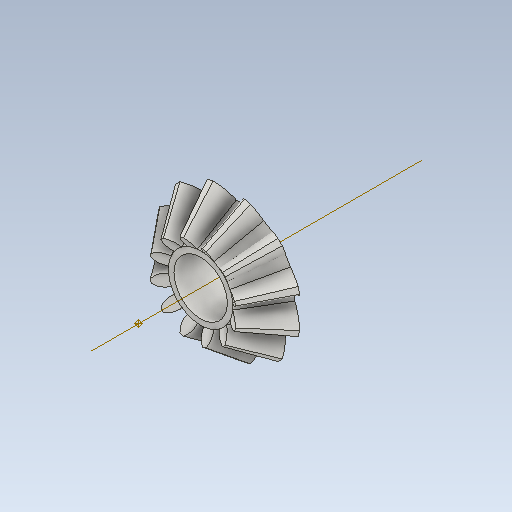
# Autodesk Inventor part: Коническая зубчатая передача12_КОПИЯ1
Saved by Autodesk Inventor 2020 (Build 240168000, 168)
## iProperties
Created: 2021-02-28
Part Number: Коническая зубчатая передача12_КОПИЯ1
Material: Steel, Mild
Document SubType Name: Modeling
Designer: Антон
Categories: <?xml version="1.0" encoding="UTF-16"?> <MemberInstance><Categories><FamilyTemplate><FamilyTemplateParameter ValueType="xs:double" Id="1" ObjectReferenceKey="da_z" ObjectType="kUserParameterObject"/><FamilyTemplateParameter ValueType="xs:double" Id="2" ObjectReferenceKey="da_b" ObjectType="kUserParameterObject"/><FamilyTemplateParameter ValueType="xs:double" Id="3" ObjectReferenceKey="da_beta" ObjectType="kUserParameterObject"/><FamilyTemplateParameter ValueType="xs:double" Id="4" ObjectReferenceKey="da_dae" ObjectType="kUserParameterObject"/><FamilyTemplateParameter ValueType="xs:double" Id="5" ObjectReferenceKey="da_ve" ObjectType="kUserParameterObject"/><FamilyTemplateParameter ValueType="xs:double" Id="6" ObjectReferenceKey="da_omega" ObjectType="kUserParameterObject"/><FamilyTemplateParameter ValueType="xs:string" Id="7" ObjectReferenceKey="EAIAABAAAAAAHwAAAAAAAIAAAAAAAAAA" ObjectType="83914240" SubObjectId="SurfaceGeometry"/></FamilyTemplate><ParamToTemplateMap><ParamToTemplate CategoryParameter="//CategoryParameter[@InternalName='046C89C9-8512-4d59-83FE-43B91F4F132A']" TemplateParameter="1"/><ParamToTemplate CategoryParameter="//CategoryParameter[@InternalName='2552DF32-E462-4b46-AEBF-C6C7768E72AC']" TemplateParameter="2"/><ParamToTemplate CategoryParameter="//CategoryParameter[@InternalName='C9EE641D-15FC-4fae-A226-E94C4372FDD7']" TemplateParameter="3"/><ParamToTemplate><ParamToTemplate CategoryParameter="//CategoryParameter[@InternalName='00B6519A-459B-49c7-AD84-2E56D39A5744']" ConstantValue="0.000000"/></ParamToTemplate><ParamToTemplate><ParamToTemplate CategoryParameter="//CategoryParameter[@InternalName='04B31F0E-C7A6-4894-AA32-9629BEFACF47']" ConstantValue="1.000000"/></ParamToTemplate><ParamToTemplate><ParamToTemplate CategoryParameter="//CategoryParameter[@InternalName='43CBEC2E-7847-49e7-A936-2F7889FCB2D9']" ConstantValue="0.200000"/></ParamToTemplate><ParamToTemplate><ParamToTemplate CategoryParameter="//CategoryParameter[@InternalName='B1EFC894-105D-4ebd-86BF-FA20ED196853']" ConstantValue="0.300000"/></ParamToTemplate><ParamToTemplate><ParamToTemplate CategoryParameter="//CategoryParameter[@InternalName='51175063-3D10-4879-93E8-6246FE8B403D']" ConstantValue="2060000000.000000"/></ParamToTemplate><ParamToTemplate><ParamToTemplate CategoryParameter="//CategoryParameter[@InternalName='A3A52E27-4454-46a9-B0BD-C932399B70AF']" ConstantValue="0.300000"/></ParamToTemplate><ParamToTemplate CategoryParameter="//CategoryParameter[@InternalName='2A200944-5A8C-41ca-B96E-8520D2E510F1']" TemplateParameter="4"/><ParamToTemplate><ParamToTemplate CategoryParameter="//CategoryParameter[@InternalName='1A637F62-92C8-44bc-B81F-10802510B579']" ConstantValue="0.818045"/></ParamToTemplate><ParamToTemplate CategoryParameter="//CategoryParameter[@InternalName='B52DD4BE-6863-48fb-BF58-89EF6F9EC65C']" TemplateParameter="5"/><ParamToTemplate><ParamToTemplate CategoryParameter="//CategoryParameter[@InternalName='3956BFF2-84D2-457d-93C2-9B0613DEBA67']" ConstantValue="0.510523"/></ParamToTemplate><ParamToTemplate CategoryParameter="//CategoryParameter[@InternalName='739CFA02-461B-4bf8-8049-181FCAD8B28F']" TemplateParameter="6"/><ParamToTemplate><ParamToTemplate CategoryParameter="//CategoryParameter[@InternalName='A27E999F-E2CE-4481-8A2A-EBF499C4C3C5']" ConstantValue="0.000000"/></ParamToTemplate><ParamToTemplate><ParamToTemplate CategoryParameter="//CategoryParameter[@InternalName='9E1B4470-B2D3-4ff1-B813-535BB4CDF51A']" ConstantValue="3520000.000000"/></ParamToTemplate><ParamToTemplate><ParamToTemplate CategoryParameter="//CategoryParameter[@InternalName='F8452263-BFF6-458c-9FB1-07C4B99E95CD']" ConstantValue="11400000.000000"/></ParamToTemplate><ParamToTemplate><ParamToTemplate CategoryParameter="//CategoryParameter[@InternalName='3E3BB259-FD49-497f-8171-6EBC954A3479']" ConstantValue="2.000000"/></ParamToTemplate><ParamToTemplate CategoryParameter="//CategoryParameter[@InternalName='27C3BAF2-7550-4e4b-AE2C-0DB134B7D9B7']" TemplateParameter="7"/></ParamToTemplateMap><Category DisplayName="Gear" InternalName="DC85795E-93AB-48d5-8EEE-5A27447B64BD" Mnemonic="Gear"><CategoryParameter DisplayName="z" InternalName="046C89C9-8512-4d59-83FE-43B91F4F132A" Mnemonic="z"/><CategoryParameter DisplayName="b" InternalName="2552DF32-E462-4b46-AEBF-C6C7768E72AC" Mnemonic="b"/><CategoryParameter DisplayName="||b|" InternalName="C9EE641D-15FC-4fae-A226-E94C4372FDD7" Mnemonic="beta"/><CategoryParameter DisplayName="x" InternalName="00B6519A-459B-49c7-AD84-2E56D39A5744" Mnemonic="x"/><CategoryParameter DisplayName="a*" InternalName="04B31F0E-C7A6-4894-AA32-9629BEFACF47" Mnemonic="a"/><CategoryParameter DisplayName="c*" InternalName="43CBEC2E-7847-49e7-A936-2F7889FCB2D9" Mnemonic="c"/><CategoryParameter DisplayName="r|.f|*" InternalName="B1EFC894-105D-4ebd-86BF-FA20ED196853" Mnemonic="rf"/><CategoryParameter DisplayName="E" InternalName="51175063-3D10-4879-93E8-6246FE8B403D" Mnemonic="E"/><CategoryParameter DisplayName="||m|" InternalName="A3A52E27-4454-46a9-B0BD-C932399B70AF" Mnemonic="mi"/><Category DisplayName="BevelGear" InternalName="0C98F69A-0C2B-4791-B2FE-7691BB227E77" Mnemonic="BevelGear"><CategoryParameter DisplayName="d|.ae|" InternalName="2A200944-5A8C-41ca-B96E-8520D2E510F1" Mnemonic="dae"/><CategoryParameter DisplayName="d|.ai|" InternalName="1A637F62-92C8-44bc-B81F-10802510B579" Mnemonic="dai"/><CategoryParameter DisplayName="J|.e|" InternalName="B52DD4BE-6863-48fb-BF58-89EF6F9EC65C" Mnemonic="ve"/><CategoryParameter DisplayName="J|.i|" InternalName="3956BFF2-84D2-457d-93C2-9B0613DEBA67" Mnemonic="vi"/><CategoryParameter DisplayName="||S|" InternalName="739CFA02-461B-4bf8-8049-181FCAD8B28F" Mnemonic="omega"/><CategoryParameter DisplayName="x|.t|" InternalName="A27E999F-E2CE-4481-8A2A-EBF499C4C3C5" Mnemonic="xt"/><CategoryParameter DisplayName="||s||.Flim|" InternalName="9E1B4470-B2D3-4ff1-B813-535BB4CDF51A" Mnemonic="sFlim"/><CategoryParameter DisplayName="||s||.Hlim|" InternalName="F8452263-BFF6-458c-9FB1-07C4B99E95CD" Mnemonic="sHlim"/><CategoryParameter DisplayName="тип" InternalName="3E3BB259-FD49-497f-8171-6EBC954A3479" Mnemonic="type"/><CategoryParameter DisplayName="PitchDiameter" InternalName="27C3BAF2-7550-4e4b-AE2C-0DB134B7D9B7" Mnemonic="IDS_PITCHDIAM"/></Category></Category></Categories></MemberInstance>
Mass: 60.9118 g
Surface Area: 34.3074 cm^2
Volume: 7.7496 cm^3
Density: 7.85 g/cm^3
Appearance: С умеренной полировкой
CustomPartVersion: 1
Author: Антон
d48: 0.000 мм
d49: 0.000 мм
d50: 90.00 град
d52: 0.000 мм
d53: 0.000 мм
d54: 0.00 град
Autodesk Inventor part; units mm, degrees
ref_plane "Плоскость сетки 2" through (0, 0, 0) normal (0.9659258, 0.258819, 0) x (0, 0, 1)
sketch "Эскиз тела зубьев" plane through (0, 0, 0) normal (1, 0, 0) x (0, 1, 0)
  line L0 (0, 0) -> (5.00154, -9.66564) construction
  line L1 (5.00154, -9.66564) -> (6.789153, -8.473898)
  line L2 (6.789153, -8.473898) -> (0, 0) construction
  line L3 (6, -9) -> (0, 0) construction
  line L4 (3.013252, -5.823209) -> (4.090226, -5.105226)
  line L5 (5.00154, -9.66564) -> (3.013252, -5.823209)
  line L6 (6.789153, -8.473898) -> (4.090226, -5.105226)
  line L7 (0, -11.598768) -> (0, 1.933128)
  line L8 (0, -9) -> (6.789153, -9) construction
  dimension "d0" = 12
  dimension "d1" = 10.00308
  dimension "d2" = 13.57831
  dimension "d3" = 4.3
  dimension "d4" = 8.4739
  constraints: 16 end point, 4 point on line, 3 perpendicular, 2 collinear, 1 horizontal alignment, 1 vertical alignment
  measures "d0" diameter of L3.start L7
  measures "d1" diameter of L0.end L7
  measures "d2" diameter of L1.end L7
  measures "d3" distance between parallel lines of L1 L4
  measures "d4" vertical distance of L1.end L0.start
revolve "Тело зубьев" add sketch "Эскиз тела зубьев" angle 360 about axis through (0, 0, 0) along (0, 0, 1)
ref_plane "Плоскость зуба" through (0, 6, -9) normal (0, -0.5547002, 0.8320503) x (1, 0, 0)
sketch "Создать эскиз" plane through (0, 6, -9) normal (0, -0.5547002, 0.8320503) x (1, 0, 0)
  line L0 (0, -8.971918) -> (0, 3.353794)
  arc A0 (-0.498934, -1.457813) -> (-2.317762, 1.282413) centre (-3.209049, -1.282917) ccw
  arc A1 (2.317762, 1.282413) -> (0.498934, -1.457813) centre (3.209049, -1.282917) ccw
  line L1 (-0.498934, -1.457813) -> (0.498934, -1.457813)
  arc A2 (2.317762, 1.282413) -> (-2.317762, 1.282413) centre (0, -7.211102) ccw
  dimension "d7" = 2.71575
  dimension "d8" = 3.20905
  dimension "d9" = 5.92819
  dimension "d57" = 8.80408
  dimension "d58" = 5.75329
  constraints: 6 point on circle, 3 centre point, 3 symmetric about line, 2 end point, 1 coincident, 1 perpendicular, 1 other
  measures "d7" radius of A0
  measures "d8" horizontal distance of point (0, -7.211) A0.centre
  measures "d9" vertical distance of point (0, -7.211) A0.centre
  measures "d57" radius of A2
  measures "d58" distance from line of A2.centre L1
ref_plane "Конечная плоскость" through (0, 3.555202, -5.332803) normal (0, -0.5547002, 0.8320503) x (1, 0, 0)
sketch "Конечный эскиз" plane through (0, 3.555202, -5.332803) normal (0, -0.5547002, 0.8320503) x (1, 0, 0)
  line L0 (0, -6.809181) -> (0, 2.545341)
  arc A0 (-0.295635, -0.863803) -> (-1.373352, 0.759873) centre (-1.90147, -0.760172) ccw
  arc A1 (1.373352, 0.759873) -> (0.295635, -0.863803) centre (1.90147, -0.760172) ccw
  line L1 (-0.295635, -0.863803) -> (0.295635, -0.863803)
  arc A2 (1.373352, 0.759873) -> (-1.373352, 0.759873) centre (0, -4.272821) ccw
  dimension "d12" = 1.60917
  dimension "d15" = 1.90147
  dimension "d16" = 3.51265
  dimension "d59" = 5.21671
  dimension "d60" = 3.40902
  constraints: 6 point on circle, 3 centre point, 3 symmetric about line, 2 end point, 1 coincident, 1 other
  measures "d12" radius of A0
  measures "d15" horizontal distance of A0.centre point (0, -4.273)
  measures "d16" vertical distance of A0.centre point (0, -4.273)
  measures "d59" radius of A2
  measures "d60" distance from line of A2.centre L1
loft "Loft" cut profiles "Создать эскиз", "Конечный эскиз"
pattern_circular "Circular Pattern" count 12 over 360 about axis through (0, 0, 0) along (0, 0, 1) of "Loft"
sketch3d "3D эскиз: справа"
ref_plane "Конечная плоскость: справа" through (-0.370626, 3.535831, -5.332803) normal (0.0578269, -0.5516778, 0.8320503) x (0.9945512, 0.104249, 0)
sketch "Конечный эскиз: справа" plane through (-0.370626, 3.535831, -5.332803) normal (0.0578269, -0.5516778, 0.8320503) x (0.9945512, 0.104249, 0)
  arc A0 (-0.295635, -0.863803) -> (-1.373352, 0.759873) centre (-1.90147, -0.760172) ccw
  line L0 (0, -7.397473) -> (0, 3.133632)
  arc A1 (1.373352, 0.759873) -> (0.295635, -0.863803) centre (1.90147, -0.760172) ccw
  line L1 (-0.295635, -0.863803) -> (0.295635, -0.863803)
  arc A2 (1.373352, 0.759873) -> (-1.373352, 0.759873) centre (0, -4.272821) ccw
  dimension "d70" = 1.90147
  dimension "d71" = 3.51265
  dimension "d72" = 1.60917
  dimension "d73" = 3.40902
  dimension "d74" = 5.21671
  constraints: 6 point on circle, 3 centre point, 3 symmetric about line, 2 end point, 1 coincident, 1 perpendicular, 1 other
  measures "d70" horizontal distance of A2.centre A0.centre
  measures "d71" vertical distance of point (0, -4.273) A0.centre
  measures "d72" radius of A0
  measures "d73" distance from line of point (0, -4.273) L1
  measures "d74" radius of A2
feature "Лофт: справа" [suppressed]
pattern_circular "Круговой массив: справа" [suppressed]
sketch3d "3D эскиз: слева"
ref_plane "Конечная плоскость: cлева" through (0.453249, 3.535831, -5.342096) normal (-0.0705746, -0.550558, 0.8318084) x (0.9918839, -0.127147, 0)
sketch "Конечный эскиз: слева" plane through (0.453249, 3.535831, -5.342096) normal (-0.0705746, -0.550558, 0.8318084) x (0.9918839, -0.127147, 0)
  line L0 (0, -11.323649) -> (0, 4.577436)
  arc A0 (-0.295635, -0.866597) -> (-1.373352, 0.757079) centre (-1.90147, -0.762966) ccw
  arc A1 (1.373352, 0.757079) -> (0.295635, -0.866597) centre (1.90147, -0.762966) ccw
  line L1 (-0.295635, -0.866597) -> (0.295635, -0.866597)
  ellipse E0 centre (0, -2.833721) end of major axis (4.090226, -2.833721) minor radius 3.402284
  arc A2 (1.373352, 0.757079) -> (-1.373352, 0.757079) centre (0, -4.275615) ccw
  dimension "d56" = 3.40228
  dimension "d30" = 1.60917
  dimension "d31" = 1.90147
  dimension "d32" = 3.51265
  dimension "d61" = 5.21671
  dimension "d62" = 3.40902
  constraints: 6 point on circle, 3 centre point, 3 symmetric about line, 2 end point, 1 coincident, 2 other
  measures "d30" radius of A0
  measures "d31" horizontal distance of point (0, -4.276) A0.centre
  measures "d32" vertical distance of A0.centre point (0, -4.276)
  measures "d61" radius of A2
  measures "d62" distance from line of point (0, -4.276) L1
feature "Лофт: слева" [suppressed]
pattern_circular "Круговой массив: слева" [suppressed]
sketch "Эскиз тела" plane through (0, 0, 0) normal (1, 0, 0) x (0, 1, 0)
  line L0 (0, -10.112435) -> (0, -6.984874)
  line L1 (5.00154, -9.66564) -> (3.013252, -5.823209)
  line L2 (3.013252, -5.823209) -> (0, -5.823209)
  line L3 (5.00154, -9.66564) -> (0, -9.66564)
  constraints: 4 end point, 2 perpendicular, 2 point on line
sketch "Эскиз тела outline for Фиксировать тело" plane through (0, 0, 0) normal (1, 0, 0) x (0, 1, 0)
  line L0 (0, -9.66564) -> (5.00154, -9.66564)
  line L1 (0, -5.823209) -> (0, -9.66564)
  line L2 (3.013252, -5.823209) -> (0, -5.823209)
  line L3 (5.00154, -9.66564) -> (3.013252, -5.823209)
revolve "Фиксировать тело" add sketch "Эскиз тела outline for Фиксировать тело" angle 360 about axis through (0, 0, 0) along (0, 0, 1)
sketch "Sketch6" plane through (0, 0, 0) normal (1, 0, 0) x (0, 1, 0)
  line L0 (6, -9) -> (0, 0) projected
  line L1 (0, -10.8) -> (0, 1.8) projected
surface revolve "Средний диаметр" sketch "Sketch6" angle 360 about axis through (0, 0, 0) along (0, 0, 1) shown no curves L0
hole "Отверстие1" at (0, 0, 0) direction (0, 0, -1) diameter 5 end through all
equation "\"d0\" = da_de"
equation "\"d1\" = da_dfe"
equation "\"d2\" = da_dae"
equation "\"d3\" = da_b"
equation "\"d4\" = da_ve"
equation "\"d7\" = fd_rr"
equation "\"d8\" = fd_x"
equation "\"d9\" = fd_y"
equation "\"d57\" = 0.5 * fd_dva + 0.3 * da_he"
equation "\"d58\" = 0.5 * fd_dva - 1.12 * da_he"
equation "\"da_teethtype\" = 0"
equation "\"da_b\" = 4.3"
equation "\"da_de\" = 12"
equation "\"da_dae\" = 13.57831"
equation "\"da_dfe\" = 10.00308"
equation "\"da_le\" = 10.81665"
equation "\"da_omega\" = 90deg"
equation "\"da_beta\" = 0"
equation "\"da_delta\" = 33.690068deg"
equation "\"da_alpha\" = 20deg"
equation "\"da_he\" = 2.14844"
equation "\"da_ve\" = 8.4739"
equation "\"da_zv\" = 14.422205"
equation "\"fd_loft\" = da_b + 0.05 * da_he"
equation "\"fd_x\" = fd_x1 + fd_x2"
equation "\"fd_y\" = fd_y1 - fd_y2"
equation "\"fd_dd\" = fd_dva - 0.8 * da_he"
equation "\"da_dvw\" = 14.42221"
equation "\"d11\" = fd_loft"
equation "\"da_dm\" = 9.61479"
equation "\"da_x\" = 0"
equation "\"da_m\" = 1"
equation "\"d50\" = da_omega"
equation "\"fd_rr\" = 2.715753"
equation "\"fd_dva\" = 16.319093"
equation "\"fd_x1\" = 0.792521"
equation "\"fd_x2\" = 2.416528"
equation "\"fd_y1\" = 7.16742"
equation "\"fd_y2\" = 1.239235"
body "Solid1"
body "Srf1"
